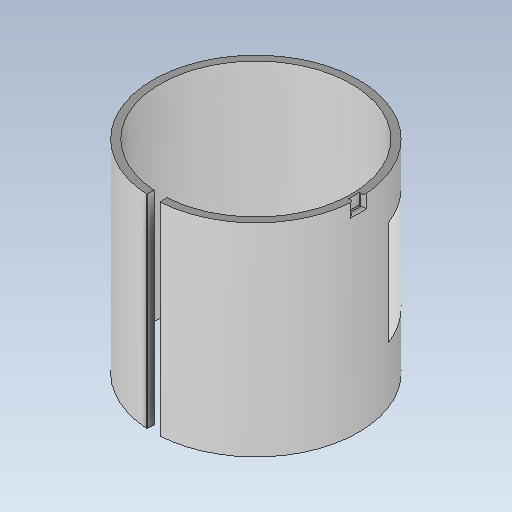
# Autodesk Inventor part: 555_Outer
Saved by Autodesk Inventor 2021 (Build 250183000, 183)
## iProperties
Created: 2021-08-07
Part Number: 555_Outer
Material: 鉄、鋳鉄
Document SubType Name: Modeling
Designer: Hagihara Yuya
Density: 7.15 g/cm^3
Appearance: アルミニウム - つや出し
Author: Hagihara Yuya
Autodesk Inventor part; units mm, degrees
ref_plane "YZ Plane" through (0, 0, 0) normal (1, 0, 0) x (0, 1, 0)
ref_plane "XZ Plane" through (0, 0, 0) normal (0, 1, 0) x (-1, 0, 0)
ref_plane "XY Plane" through (0, 0, 0) normal (0, 0, 1) x (1, 0, 0)
sketch "スケッチ1" plane through (0, 0, 0) normal (0, 0, 1) x (1, 0, 0)
  circle A0 centre (0, 0) radius 17.9
  circle A1 centre (0, 0) radius 19.25
  line L0 (0, 0) -> (1.25, 19.2094)
  line L1 (0, 0) -> (-1.25, 19.2094)
  line L2 (0, -26.95) -> (0, 26.95) projected
  point P0 (1.1623, 17.8622)
  point P1 (-1.1623, 17.8622)
  dimension "d0" = 35.8
  dimension "d1" = 38.5
  dimension "d4" = 2.5
  constraints: 4 end point, 2 centre point, 2 coincident, 2 point on circle, 1 other
  measures "d0" diameter of A0
  measures "d1" diameter of A1
  measures "d4" distance of L0.end L1.end
extrude "押し出し1" add sketch "スケッチ1" along normal blind 38 contours A0 L0 A1 L2 | L2 A1 L1 A0 picked at (1.4278, -18.6391) picked at (-2.7104, 18.4842)
sketch "スケッチ2" plane through (0, 0, 38) normal (0, 0, 1) x (1, 0, 0)
  line L0 (0, 0) -> (-19.224, -1)
  arc A0 (-1.25, 19.2094) -> (1.25, 19.2094) centre (0, 0) ccw projected
  line L1 (0, 0) -> (-19.224, 1)
  line L2 (-26.95, 0) -> (26.95, 0) projected
  arc A1 (-18.3752, 0.9558) -> (-18.3752, -0.9558) centre (0, 0) ccw
  arc A2 (-1.1623, 17.8622) -> (1.1623, 17.8622) centre (0, 0) ccw projected
  dimension "d5" = 2
  dimension "d6" = 0.5
  constraints: 4 end point, 4 point on circle, 2 point on line, 1 centre point, 1 coincident, 1 other
  measures "d5" distance of L0.end L1.end
  measures "d6" radial gap between concentric circles of A1 A2
extrude "押し出し2" cut sketch "スケッチ2" against normal blind 2 contours L0 A0 L2 A1 | L2 A0 L1 A1
fillet "フィレット1" radius 0.5 3 edges at (-19.25, 0, 36) (-19.224, -1, 37) (-19.224, 1, 37)
sketch "スケッチ3" plane through (0, 0, 0) normal (0, 1, 0) x (-1, 0, 0)
  line L0 (-18, 30) -> (18, 30)
  line L1 (18, 30) -> (18, 10.5)
  line L2 (18, 10.5) -> (-18, 10.5)
  line L3 (-18, 10.5) -> (-18, 30)
  line L4 (19.1905, 38) -> (-19.25, 38) projected
  point P0 (0, 0)
  point P1 (-1.25, 38)
  point P2 (0, 10.5)
  dimension "d10" = 8
  dimension "d11" = 19.5
  dimension "d12" = 36
  constraints: 8 end point, 2 parallel, 1 horizontal, 1 midpoint, 1 perpendicular, 1 vertical alignment
  measures "d10" distance between parallel lines of L4 L0
  measures "d11" distance between parallel lines of L2 L0
  measures "d12" distance of L1.end L2.end
sketch3d "3D スケッチ1"
split_face "分割1"
fillet "フィレット2" radius 0.1 2 edges at (-1.25, 19.2094, 19) (1.25, 19.2094, 19)
